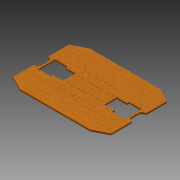
# Autodesk Inventor part: Chassis
Saved by Autodesk Inventor 2014 SP1 (Build 180222100, 222)
## iProperties
Created: 2015-03-16
Part Number: Chassis
Material: Wood (Oak)
Document SubType Name: Modeling
Designer: david
Density: 0.76 g/cm^3
Appearance: White Oak - Natural Medium Gloss
Mass: 340.731 g
Surface Area: 1620.88 cm^2
Volume: 448.331 cm^3
Author: david
Autodesk Inventor part; units mm, degrees
ref_plane "YZ Plane" through (0, 0, 0) normal (1, 0, 0) x (0, 1, 0)
ref_plane "XZ Plane" through (0, 0, 0) normal (0, 1, 0) x (-1, 0, 0)
ref_plane "XY Plane" through (0, 0, 0) normal (0, 0, 1) x (1, 0, 0)
sketch "BodySketch" plane through (0, 0, 0) normal (0, 1, 0) x (-1, 0, 0)
  line L0 (0, 125) -> (125, 125)
  line L1 (125, 125) -> (175, 100)
  line L2 (175, 100) -> (175, 24.5)
  line L3 (175, 24.5) -> (169, 24.5)
  line L4 (160.5, 18) -> (160.5, -18)
  line L5 (169, -24.5) -> (175, -24.5)
  line L6 (175, -24.5) -> (175, -100)
  line L7 (175, -100) -> (125, -125)
  line L8 (125, -125) -> (0, -125)
  line L9 (0, 0) -> (0, 145.614) construction
  line L10 (0, 125) -> (-125, 125)
  line L11 (-125, 125) -> (-175, 100)
  line L12 (-175, 100) -> (-175, 24.5)
  line L13 (-175, -24.5) -> (-175, -100)
  line L14 (-175, -100) -> (-125, -125)
  line L15 (-125, -125) -> (0, -125)
  line L16 (0, 0) -> (316.974, 0) construction
  line L17 (160.5, 18) -> (169, 24.5)
  line L18 (160.5, -18) -> (169, -24.5)
  line L19 (-175, 24.5) -> (-169, 24.5)
  line L20 (-160.5, 18) -> (-160.5, -18)
  line L21 (-169, -24.5) -> (-175, -24.5)
  line L22 (-160.5, 18) -> (-169, 24.5)
  line L23 (-160.5, -18) -> (-169, -24.5)
  point P0 (160.5, 24.5)
  point P1 (160.5, -24.5)
  dimension "Chassis_Body_Width" = 350
  dimension "Chassis_Body_Length" = 250
  dimension "Chassis_EncoderWheelSpace_Diameter" = 49
  dimension "Chassis_EncoderWheelSpace_Width" = 14.5
  dimension "Chassis_Body_InnerLength" = 200
  dimension "Chassis_Body_InnerWidth" = 250
  dimension "d14" = 6
  dimension "d15" = 36
  constraints: 48 end point, 12 symmetric about line, 5 parallel, 2 collinear, 2 equal length, 2 perpendicular, 2 point on line, 1 horizontal, 2 other
  measures "Chassis_Body_Width" distance between parallel lines of L2 L12
  measures "Chassis_Body_Length" distance between parallel lines of L8 L0
  measures "Chassis_EncoderWheelSpace_Diameter" distance between parallel lines of L5 L3
  measures "Chassis_EncoderWheelSpace_Width" distance between parallel lines of L2 L4
  measures "Chassis_Body_InnerLength" distance of L6.end L1.end
  measures "Chassis_Body_InnerWidth" distance of L0.end L10.end
  measures "d14" distance of L3.end L2.end
  measures "d15" distance of L4.start L4.end
extrude "Body" add sketch "BodySketch" along normal blind 6
sketch "EncoderBodyHoleSketch" plane through (0, 6, 0) normal (0, 1, 0) x (1, 0, 0)
  line L0 (-175, 100) -> (-175, 24.5) projected
  line L1 (-175, -24.5) -> (-175, -100) projected
  line L2 (0, 0) -> (0, 145.3586) construction
  line L3 (-154.5, 30.25) -> (-109.5, 30.25)
  line L4 (-109.5, 30.25) -> (-109.5, -30.25)
  line L5 (-109.5, -30.25) -> (-154.5, -30.25)
  line L6 (-154.5, -30.25) -> (-154.5, 30.25)
  line L7 (0, 0) -> (187.4589, 0) construction
  line L8 (154.5, 30.25) -> (109.5, 30.25)
  line L9 (109.5, 30.25) -> (109.5, -30.25)
  line L10 (109.5, -30.25) -> (154.5, -30.25)
  line L11 (154.5, -30.25) -> (154.5, 30.25)
  line L12 (-169, -24.5) -> (-175, -24.5) projected
  line L13 (-132, 0) -> (-132, 72.6793) construction
  point P0 (-160.5, -24.5)
  dimension "d9" = 45
  dimension "d10" = 60.5
  dimension "d13" = 43
  constraints: 22 end point, 4 parallel, 4 symmetric about line, 3 perpendicular, 1 horizontal, 2 other
  measures "d9" distance between parallel lines of L4 L6
  measures "d10" distance between parallel lines of L5 L3
  measures "d13" distance between parallel lines of L13 L0
extrude "EncoderBodyHole" cut sketch "EncoderBodyHoleSketch" against normal up to next
sketch "EncoderSupportFasteningSketch" plane through (0, 6, 0) normal (0, 1, 0) x (1, 0, 0)
  line L0 (-175, 100) -> (-175, 24.5) projected
  line L1 (-175, -24.5) -> (-175, -100) projected
  line L2 (0, 0) -> (0, 103.2036) construction
  line L3 (-120.5, 39.75) -> (-153.5, 39.75) construction
  line L4 (-153.5, 39.75) -> (-153.5, -39.75) construction
  line L5 (-153.5, -39.75) -> (-120.5, -39.75) construction
  line L6 (-120.5, -39.75) -> (-120.5, 39.75) construction
  line L7 (0, 0) -> (196.594, 0) construction
  circle A0 centre (-148.5, 34.75) radius 1.5
  circle A1 centre (-148.5, -34.75) radius 1.5
  line L8 (-137, 47.3947) -> (-137, -51.0004) construction
  circle A2 centre (-125.5, 34.75) radius 1.5
  circle A3 centre (-125.5, -34.75) radius 1.5
  circle A4 centre (148.5, 34.75) radius 1.5
  circle A5 centre (148.5, -34.75) radius 1.5
  circle A6 centre (125.5, 34.75) radius 1.5
  circle A7 centre (125.5, -34.75) radius 1.5
  dimension "d16" = 79.5
  dimension "d17" = 33
  dimension "d18" = 21.5
  dimension "d19" = 3
  dimension "d20" = 5
  dimension "d21" = 5
  dimension "d22" = 16.5
  constraints: 14 end point, 8 centre point, 7 symmetric about line, 3 parallel, 3 perpendicular, 1 horizontal, 8 other
  measures "d16" distance between parallel lines of L5 L3
  measures "d17" distance between parallel lines of L4 L6
  measures "d18" distance between parallel lines of L0 L4
  measures "d19" diameter of A0
  measures "d20" distance from line of L3 A0.centre
  measures "d21" distance from line of L4 A0.centre
  measures "d22" distance between parallel lines of L4 L8
extrude "EncoderSupportFastening" cut sketch "EncoderSupportFasteningSketch" against normal up to next
sketch "MotorBlockFasteningSketch" plane through (0, 6, 0) normal (0, 1, 0) x (1, 0, 0)
  line L0 (10.676, -18) -> (24.3135, -18) construction
  circle A0 centre (7.5, -18) radius 1.5
  circle A1 centre (22.5, -18) radius 1.5
  line L1 (0, 0) -> (0, -28.6489) construction
  circle A2 centre (46.5, -18) radius 1.5
  circle A3 centre (61.5, -18) radius 1.5
  circle A4 centre (7.5, -46) radius 1.5
  circle A5 centre (22.5, -46) radius 1.5
  circle A6 centre (46.5, -46) radius 1.5
  circle A7 centre (61.5, -46) radius 1.5
  circle A8 centre (-7.5, -18) radius 1.5
  circle A9 centre (-22.5, -18) radius 1.5
  circle A10 centre (-46.5, -18) radius 1.5
  circle A11 centre (-61.5, -18) radius 1.5
  circle A12 centre (-7.5, -46) radius 1.5
  circle A13 centre (-22.5, -46) radius 1.5
  circle A14 centre (-46.5, -46) radius 1.5
  circle A15 centre (-61.5, -46) radius 1.5
  line L2 (0, 0) -> (72.0385, 0) construction
  circle A16 centre (7.5, 18) radius 1.5
  circle A17 centre (22.5, 18) radius 1.5
  line L3 (0, 0) -> (0, 28.6489) construction
  circle A18 centre (46.5, 18) radius 1.5
  circle A19 centre (61.5, 18) radius 1.5
  circle A20 centre (7.5, 46) radius 1.5
  circle A21 centre (22.5, 46) radius 1.5
  circle A22 centre (46.5, 46) radius 1.5
  circle A23 centre (61.5, 46) radius 1.5
  circle A24 centre (-7.5, 18) radius 1.5
  circle A25 centre (-22.5, 18) radius 1.5
  circle A26 centre (-46.5, 18) radius 1.5
  circle A27 centre (-46.5, 46) radius 1.5
  circle A28 centre (-61.5, 18) radius 1.5
  circle A29 centre (-61.5, 46) radius 1.5
  circle A30 centre (-7.5, 46) radius 1.5
  circle A31 centre (-22.5, 46) radius 1.5
  dimension "d25" = 3
  dimension "d28" = 15
  dimension "d35" = 39
  dimension "d38" = 28
  dimension "d41" = 15
  dimension "d46" = 18
  constraints: 32 centre point, 25 symmetric about line, 8 end point, 3 horizontal, 1 perpendicular, 1 point on line, 1 vertical, 38 other
  measures "d25" diameter of A0
  measures "d28" distance of A0.centre A1.centre
  measures "d35" distance of A0.centre A2.centre
  measures "d38" distance of A0.centre A4.centre
  measures "d41" distance of A0.centre A8.centre
  measures "d46" distance between parallel lines of L2 L0
extrude "MotorBlockFastening" cut sketch "MotorBlockFasteningSketch" against normal up to next
sketch "MotorWheelHoleSketch" plane through (0, 6, 0) normal (0, 1, 0) x (1, 0, 0)
  line L0 (-109.5, 30.25) -> (-109.5, -30.25) projected
  line L1 (-109.5, 22.5) -> (-73.5, 22.5)
  line L2 (-73.5, 22.5) -> (-73.5, -22.5)
  line L3 (-73.5, -22.5) -> (-109.5, -22.5)
  line L4 (-109.5, -22.5) -> (-109.5, 22.5)
  line L5 (0, 0) -> (72.3504, 0) construction
  line L6 (-175, -24.5) -> (-175, -100) projected
  line L7 (0, 0) -> (0, 70.7306) construction
  line L8 (109.5, 22.5) -> (73.5, 22.5)
  line L9 (73.5, 22.5) -> (73.5, -22.5)
  line L10 (73.5, -22.5) -> (109.5, -22.5)
  line L11 (109.5, -22.5) -> (109.5, 22.5)
  dimension "d49" = 36
  dimension "d50" = 45
  constraints: 20 end point, 4 symmetric about line, 3 parallel, 2 perpendicular, 1 horizontal, 1 point on line, 1 other
  measures "d49" distance between parallel lines of L2 L4
  measures "d50" distance between parallel lines of L3 L1
extrude "MotorWheelHole" cut sketch "MotorWheelHoleSketch" against normal up to next
equation "\"Chassis_EncoderWheelSpace_Diameter\" = EncoderWheel_Tyre_Diameter"
equation "\"Chassis_EncoderWheelSpace_Width\" = EncoderBlock_InterfaceToWheel_Distance + Chassis_MecanicalSpace"
equation "\"d14\" = EncoderWheel_Tyre_Width"
equation "\"d15\" = EncoderWheelInterface_Diameter"
equation "\"d9\" = EncoderSupportInside_Front_Thickness + Encoder_Body_Length + 2 * Chassis_MecanicalSpace"
equation "\"d10\" = EncoderSupportInside_Width + 2 * Chassis_MecanicalSpace"
equation "\"d13\" = EncoderBlock_SupportToWheel_Distance + 0.5 * Encoder_Body_Length + 0.5 * EncoderSupportInside_Front_Thickness"
equation "\"d16\" = EncoderSupportOutside_Width"
equation "\"d17\" = EncoderSupportOutside_Length"
equation "\"d18\" = EncoderBlock_SupportToWheel_Distance"
equation "\"d19\" = EncoderSupport_FixingHole_Diameter"
equation "\"d20\" = EncoderSupport_FixingnHole_Margin"
equation "\"d21\" = EncoderSupport_FixingnHole_Margin"
equation "\"d22\" = 0.5 * EncoderSupportOutside_Length"
equation "\"d28\" = Bracket_Holes_Distance"
equation "\"d35\" = Bracket_Holes_Distance + Bracket_Holes_UnfoldedDistance"
equation "\"d38\" = Bracket_Holes_LateralDistance"
equation "\"d41\" = Bracket_Holes_Distance"
equation "\"d46\" = Motor_FasteningHole_DistanceToCenter"
equation "\"Chassis_MecanicalSpace\" = 1"
equation "\"EncoderWheel_Tyre_Diameter\" = 49"
equation "\"EncoderBlock_InterfaceToWheel_Distance\" = 13.5"
equation "\"EncoderWheel_Tyre_Width\" = 6"
equation "\"EncoderWheelInterface_Diameter\" = 36"
equation "\"EncoderSupportInside_Front_Thickness\" = 3"
equation "\"Encoder_Body_Length\" = 40"
equation "\"EncoderSupportInside_Width\" = 58.5"
equation "\"EncoderBlock_SupportToWheel_Distance\" = 21.5"
equation "\"EncoderSupportOutside_Width\" = 79.5"
equation "\"EncoderSupportOutside_Length\" = 33"
equation "\"EncoderSupport_FixingHole_Diameter\" = 3"
equation "\"EncoderSupport_FixingnHole_Margin\" = 5"
equation "\"Bracket_Holes_Distance\" = 15"
equation "\"Bracket_Holes_UnfoldedDistance\" = 24"
equation "\"Bracket_Holes_LateralDistance\" = 28"
equation "\"Motor_FasteningHole_DistanceToCenter\" = 18"
body "Solid1"
